Autodesk Fusion 360 part; units mm, degrees
note: some values were not read from the file. Chosen so that the rebuilt part matches the saved one: which bodies a step acts on; which face or edge a step refers to. Set by a fixed rule: which sketch regions a step uses.
(part 2 of 2)
sketch "Sketch5" plane through (0, 0, 0) normal (0, 0, 1) x (-1, 0, 0)
  line L0 (-11.6608, -63.9455) -> (-11.5909, -63.4815)
  line L1 (-11.5909, -63.4815) -> (-7.6356, -64.0777)
  line L2 (-7.6356, -64.0777) -> (-7.7055, -64.5417)
  arc A0 (-7.7055, -64.5417) -> (-2, -64.9692) centre (0, 0) ccw
  line L3 (-2, -64.9692) -> (-2, -64.5)
  line L4 (-2, -64.5) -> (2, -64.5)
  line L5 (2, -64.5) -> (2, -64.9692)
  arc A1 (2, -64.9692) -> (7.7055, -64.5417) centre (0, 0) ccw
  line L6 (7.7055, -64.5417) -> (7.6356, -64.0777)
  line L7 (7.6356, -64.0777) -> (11.5909, -63.4815)
  line L8 (11.5909, -63.4815) -> (11.6608, -63.9455)
  arc A2 (11.6608, -63.9455) -> (17.2389, -62.6723) centre (0, 0) ccw
  line L9 (17.2389, -62.6723) -> (17.1006, -62.224)
  line L10 (17.1006, -62.224) -> (20.9229, -61.0449)
  line L11 (20.9229, -61.0449) -> (21.0612, -61.4933)
  arc A3 (21.0612, -61.4933) -> (26.3872, -59.403) centre (0, 0) ccw
  line L12 (26.3872, -59.403) -> (26.1836, -58.9803)
  line L13 (26.1836, -58.9803) -> (29.7874, -57.2447)
  line L14 (29.7874, -57.2447) -> (29.991, -57.6675)
  arc A4 (29.991, -57.6675) -> (34.946, -54.8067) centre (0, 0) ccw
  line L15 (34.946, -54.8067) -> (34.6817, -54.419)
  line L16 (34.6817, -54.419) -> (37.9866, -52.1658)
  line L17 (37.9866, -52.1658) -> (38.2509, -52.5535)
  arc A5 (38.2509, -52.5535) -> (42.7242, -48.9862) centre (0, 0) ccw
  line L18 (42.7242, -48.9862) -> (42.405, -48.6422)
  line L19 (42.405, -48.6422) -> (45.3372, -45.9215)
  line L20 (45.3372, -45.9215) -> (45.6564, -46.2655)
  arc A6 (45.6564, -46.2655) -> (49.548, -42.0713) centre (0, 0) ccw
  line L21 (49.548, -42.0713) -> (49.1812, -41.7788)
  line L22 (49.1812, -41.7788) -> (51.6751, -38.6514)
  line L23 (51.6751, -38.6514) -> (52.042, -38.944)
  arc A7 (52.042, -38.944) -> (55.265, -34.2167) centre (0, 0) ccw
  line L24 (55.265, -34.2167) -> (54.8586, -33.9821)
  line L25 (54.8586, -33.9821) -> (56.8586, -30.5179)
  line L26 (56.8586, -30.5179) -> (57.265, -30.7526)
  arc A8 (57.265, -30.7526) -> (59.7475, -25.5977) centre (0, 0) ccw
  line L27 (59.7475, -25.5977) -> (59.3107, -25.4262)
  line L28 (59.3107, -25.4262) -> (60.772, -21.7027)
  line L29 (60.772, -21.7027) -> (61.2088, -21.8742)
  arc A9 (61.2088, -21.8742) -> (62.8953, -16.4069) centre (0, 0) ccw
  line L30 (62.8953, -16.4069) -> (62.4378, -16.3025)
  line L31 (62.4378, -16.3025) -> (63.3279, -12.4027)
  line L32 (63.3279, -12.4027) -> (63.7854, -12.5072)
  arc A10 (63.7854, -12.5072) -> (64.6381, -6.8496) centre (0, 0) ccw
  line L33 (64.6381, -6.8496) -> (64.1702, -6.8145)
  line L34 (64.1702, -6.8145) -> (64.4691, -2.8257)
  line L35 (64.4691, -2.8257) -> (64.937, -2.8607)
  arc A11 (64.937, -2.8607) -> (64.937, 2.8607) centre (0, 0) ccw
  line L36 (64.937, 2.8607) -> (64.4691, 2.8257)
  line L37 (64.4691, 2.8257) -> (64.1702, 6.8145)
  line L38 (64.1702, 6.8145) -> (64.6381, 6.8496)
  arc A12 (64.6381, 6.8496) -> (63.7854, 12.5072) centre (0, 0) ccw
  line L39 (63.7854, 12.5072) -> (63.3279, 12.4027)
  line L40 (63.3279, 12.4027) -> (62.4378, 16.3025)
  line L41 (62.4378, 16.3025) -> (62.8953, 16.4069)
  arc A13 (62.8953, 16.4069) -> (61.2088, 21.8742) centre (0, 0) ccw
  line L42 (61.2088, 21.8742) -> (60.772, 21.7027)
  line L43 (60.772, 21.7027) -> (59.3107, 25.4262)
  line L44 (59.3107, 25.4262) -> (59.7475, 25.5977)
  arc A14 (59.7475, 25.5977) -> (57.265, 30.7526) centre (0, 0) ccw
  line L45 (57.265, 30.7526) -> (56.8586, 30.5179)
  line L46 (56.8586, 30.5179) -> (54.8586, 33.9821)
  line L47 (54.8586, 33.9821) -> (55.265, 34.2167)
  arc A15 (55.265, 34.2167) -> (52.042, 38.944) centre (0, 0) ccw
  line L48 (52.042, 38.944) -> (51.6751, 38.6514)
  line L49 (51.6751, 38.6514) -> (49.1812, 41.7788)
  line L50 (49.1812, 41.7788) -> (49.548, 42.0713)
  arc A16 (49.548, 42.0713) -> (45.6564, 46.2655) centre (0, 0) ccw
  line L51 (45.6564, 46.2655) -> (45.3372, 45.9215)
  line L52 (45.3372, 45.9215) -> (42.405, 48.6422)
  line L53 (42.405, 48.6422) -> (42.7242, 48.9862)
  arc A17 (42.7242, 48.9862) -> (38.2509, 52.5535) centre (0, 0) ccw
  line L54 (38.2509, 52.5535) -> (37.9866, 52.1658)
  line L55 (37.9866, 52.1658) -> (34.6817, 54.419)
  line L56 (34.6817, 54.419) -> (34.946, 54.8067)
  arc A18 (34.946, 54.8067) -> (29.991, 57.6675) centre (0, 0) ccw
  line L57 (29.991, 57.6675) -> (29.7874, 57.2447)
  line L58 (29.7874, 57.2447) -> (26.1836, 58.9803)
  line L59 (26.1836, 58.9803) -> (26.3872, 59.403)
  arc A19 (26.3872, 59.403) -> (21.0612, 61.4933) centre (0, 0) ccw
  line L60 (21.0612, 61.4933) -> (20.9229, 61.0449)
  line L61 (20.9229, 61.0449) -> (17.1006, 62.224)
  line L62 (17.1006, 62.224) -> (17.2389, 62.6723)
  arc A20 (17.2389, 62.6723) -> (11.6608, 63.9455) centre (0, 0) ccw
  line L63 (11.6608, 63.9455) -> (11.5909, 63.4815)
  line L64 (11.5909, 63.4815) -> (7.6356, 64.0777)
  line L65 (7.6356, 64.0777) -> (7.7055, 64.5417)
  arc A21 (7.7055, 64.5417) -> (2, 64.9692) centre (0, 0) ccw
  line L66 (2, 64.9692) -> (2, 64.5)
  line L67 (2, 64.5) -> (-2, 64.5)
  line L68 (-2, 64.5) -> (-2, 64.9692)
  arc A22 (-2, 64.9692) -> (-7.7055, 64.5417) centre (0, 0) ccw
  line L69 (-7.7055, 64.5417) -> (-7.6356, 64.0777)
  line L70 (-7.6356, 64.0777) -> (-11.5909, 63.4815)
  line L71 (-11.5909, 63.4815) -> (-11.6608, 63.9455)
  arc A23 (-11.6608, 63.9455) -> (-17.2389, 62.6723) centre (0, 0) ccw
  line L72 (-17.2389, 62.6723) -> (-17.1006, 62.224)
  line L73 (-17.1006, 62.224) -> (-20.9229, 61.0449)
  line L74 (-20.9229, 61.0449) -> (-21.0612, 61.4933)
  arc A24 (-21.0612, 61.4933) -> (-26.3872, 59.403) centre (0, 0) ccw
  line L75 (-26.3872, 59.403) -> (-26.1836, 58.9803)
  line L76 (-26.1836, 58.9803) -> (-29.7874, 57.2447)
  line L77 (-29.7874, 57.2447) -> (-29.991, 57.6675)
  arc A25 (-29.991, 57.6675) -> (-34.946, 54.8067) centre (0, 0) ccw
  line L78 (-34.946, 54.8067) -> (-34.6817, 54.419)
  line L79 (-34.6817, 54.419) -> (-37.9866, 52.1658)
  line L80 (-37.9866, 52.1658) -> (-38.2509, 52.5535)
  arc A26 (-38.2509, 52.5535) -> (-42.7242, 48.9862) centre (0, 0) ccw
  line L81 (-42.7242, 48.9862) -> (-42.405, 48.6422)
  line L82 (-42.405, 48.6422) -> (-45.3372, 45.9215)
  line L83 (-45.3372, 45.9215) -> (-45.6564, 46.2655)
  arc A27 (-45.6564, 46.2655) -> (-49.548, 42.0713) centre (0, 0) ccw
  line L84 (-49.548, 42.0713) -> (-49.1812, 41.7788)
  line L85 (-49.1812, 41.7788) -> (-51.6751, 38.6514)
  line L86 (-51.6751, 38.6514) -> (-52.042, 38.944)
  arc A28 (-52.042, 38.944) -> (-55.265, 34.2167) centre (0, 0) ccw
  line L87 (-55.265, 34.2167) -> (-54.8586, 33.9821)
  line L88 (-54.8586, 33.9821) -> (-56.8586, 30.5179)
  line L89 (-56.8586, 30.5179) -> (-57.265, 30.7526)
  arc A29 (-57.265, 30.7526) -> (-59.7475, 25.5977) centre (0, 0) ccw
  line L90 (-59.7475, 25.5977) -> (-59.3107, 25.4262)
  line L91 (-59.3107, 25.4262) -> (-60.772, 21.7027)
  line L92 (-60.772, 21.7027) -> (-61.2088, 21.8742)
  arc A30 (-61.2088, 21.8742) -> (-62.8953, 16.4069) centre (0, 0) ccw
  line L93 (-62.8953, 16.4069) -> (-62.4378, 16.3025)
  line L94 (-62.4378, 16.3025) -> (-63.3279, 12.4027)
  line L95 (-63.3279, 12.4027) -> (-63.7854, 12.5072)
  arc A31 (-63.7854, 12.5072) -> (-64.6381, 6.8496) centre (0, 0) ccw
  line L96 (-64.6381, 6.8496) -> (-64.1702, 6.8145)
  line L97 (-64.1702, 6.8145) -> (-64.4691, 2.8257)
  line L98 (-64.4691, 2.8257) -> (-64.937, 2.8607)
  arc A32 (-64.937, 2.8607) -> (-64.937, -2.8607) centre (0, 0) ccw
  line L99 (-64.937, -2.8607) -> (-64.4691, -2.8257)
  line L100 (-64.4691, -2.8257) -> (-64.1702, -6.8145)
  line L101 (-64.1702, -6.8145) -> (-64.6381, -6.8496)
  arc A33 (-64.6381, -6.8496) -> (-63.7854, -12.5072) centre (0, 0) ccw
  line L102 (-63.7854, -12.5072) -> (-63.3279, -12.4027)
  line L103 (-63.3279, -12.4027) -> (-62.4378, -16.3025)
  line L104 (-62.4378, -16.3025) -> (-62.8953, -16.4069)
  arc A34 (-62.8953, -16.4069) -> (-61.2088, -21.8742) centre (0, 0) ccw
  line L105 (-61.2088, -21.8742) -> (-60.772, -21.7027)
  line L106 (-60.772, -21.7027) -> (-59.3107, -25.4262)
  line L107 (-59.3107, -25.4262) -> (-59.7475, -25.5977)
  arc A35 (-59.7475, -25.5977) -> (-57.265, -30.7526) centre (0, 0) ccw
  line L108 (-57.265, -30.7526) -> (-56.8586, -30.5179)
  line L109 (-56.8586, -30.5179) -> (-54.8586, -33.9821)
  line L110 (-54.8586, -33.9821) -> (-55.265, -34.2167)
  arc A36 (-55.265, -34.2167) -> (-52.042, -38.944) centre (0, 0) ccw
  line L111 (-52.042, -38.944) -> (-51.6751, -38.6514)
  line L112 (-51.6751, -38.6514) -> (-49.1812, -41.7788)
  line L113 (-49.1812, -41.7788) -> (-49.548, -42.0713)
  arc A37 (-49.548, -42.0713) -> (-45.6564, -46.2655) centre (0, 0) ccw
  line L114 (-45.6564, -46.2655) -> (-45.3372, -45.9215)
  line L115 (-45.3372, -45.9215) -> (-42.405, -48.6422)
  line L116 (-42.405, -48.6422) -> (-42.7242, -48.9862)
  arc A38 (-42.7242, -48.9862) -> (-38.2509, -52.5535) centre (0, 0) ccw
  line L117 (-38.2509, -52.5535) -> (-37.9866, -52.1658)
  line L118 (-37.9866, -52.1658) -> (-34.6817, -54.419)
  line L119 (-34.6817, -54.419) -> (-34.946, -54.8067)
  arc A39 (-34.946, -54.8067) -> (-29.991, -57.6675) centre (0, 0) ccw
  line L120 (-29.991, -57.6675) -> (-29.7874, -57.2447)
  line L121 (-29.7874, -57.2447) -> (-26.1836, -58.9803)
  line L122 (-26.1836, -58.9803) -> (-26.3872, -59.403)
  arc A40 (-26.3872, -59.403) -> (-21.0612, -61.4933) centre (0, 0) ccw
  line L123 (-21.0612, -61.4933) -> (-20.9229, -61.0449)
  line L124 (-20.9229, -61.0449) -> (-17.1006, -62.224)
  line L125 (-17.1006, -62.224) -> (-17.2389, -62.6723)
  arc A41 (-17.2389, -62.6723) -> (-11.6608, -63.9455) centre (0, 0) ccw
  arc A42 (44.2503, 36.7173) -> (-44.2503, 36.7173) centre (0, 0) ccw
  arc A43 (43.1721, 30.6989) -> (44.2503, 36.7173) centre (41.1721, 34.163) ccw
  line L126 (43.1721, 30.6989) -> (23.6426, 19.4236)
  arc A44 (18.8944, 19.9813) -> (23.6426, 19.4236) centre (21.6426, 22.8877) ccw
  arc A45 (18.8944, 19.9813) -> (-18.8944, 19.9813) centre (0, 0) ccw
  arc A46 (-23.6426, 19.4236) -> (-18.8944, 19.9813) centre (-21.6426, 22.8877) ccw
  line L127 (-23.6426, 19.4236) -> (-43.1721, 30.6989)
  arc A47 (-44.2503, 36.7173) -> (-43.1721, 30.6989) centre (-41.1721, 34.163) ccw
  arc A48 (-26.7515, 6.3723) -> (-7.8571, -26.3537) centre (0, 0) ccw
  arc A49 (-5, -30.1869) -> (-7.8571, -26.3537) centre (-9, -30.1869) ccw
  line L128 (-5, -30.1869) -> (-5, -52.7376)
  arc A50 (-9.6729, -56.6806) -> (-5, -52.7376) centre (-9, -52.7376) ccw
  arc A51 (-53.9232, 19.9633) -> (-9.6729, -56.6806) centre (0, 0) ccw
  arc A52 (-48.1721, 22.0387) -> (-53.9232, 19.9633) centre (-50.1721, 18.5746) ccw
  line L129 (-48.1721, 22.0387) -> (-28.6426, 10.7633)
  arc A53 (-26.7515, 6.3723) -> (-28.6426, 10.7633) centre (-30.6426, 7.2992) ccw
  line L130 (-2.3412, -7.1252) -> (-9.1913, -11.0801)
  arc A54 (-14.6554, -9.616) -> (-9.1913, -11.0801) centre (-11.1913, -7.616) ccw
  line L131 (-14.6554, -9.616) -> (-15.6554, -7.884)
  arc A55 (-14.1913, -2.4199) -> (-15.6554, -7.884) centre (-12.1913, -5.884) ccw
  line L132 (-14.1913, -2.4199) -> (-7.3412, 1.535)
  arc A56 (-5, 5.5902) -> (-7.3412, 1.535) centre (0, 0) ccw
  line L133 (-5, 5.5902) -> (-5, 13.5)
  arc A57 (-1, 17.5) -> (-5, 13.5) centre (-1, 13.5) ccw
  line L134 (-1, 17.5) -> (1, 17.5)
  arc A58 (5, 13.5) -> (1, 17.5) centre (1, 13.5) ccw
  line L135 (5, 13.5) -> (5, 5.5902)
  arc A59 (7.3412, 1.535) -> (5, 5.5902) centre (0, 0) ccw
  line L136 (7.3412, 1.535) -> (14.1913, -2.4199)
  arc A60 (15.6554, -7.884) -> (14.1913, -2.4199) centre (12.1913, -5.884) ccw
  line L137 (15.6554, -7.884) -> (14.6554, -9.616)
  arc A61 (9.1913, -11.0801) -> (14.6554, -9.616) centre (11.1913, -7.616) ccw
  line L138 (9.1913, -11.0801) -> (2.3412, -7.1252)
  arc A62 (-2.3412, -7.1252) -> (2.3412, -7.1252) centre (0, 0) ccw
  arc A63 (7.8571, -26.3537) -> (26.7515, 6.3723) centre (0, 0) ccw
  arc A64 (28.6426, 10.7633) -> (26.7515, 6.3723) centre (30.6426, 7.2992) ccw
  line L139 (28.6426, 10.7633) -> (48.1721, 22.0387)
  arc A65 (53.9232, 19.9633) -> (48.1721, 22.0387) centre (50.1721, 18.5746) ccw
  arc A66 (9.6729, -56.6806) -> (53.9232, 19.9633) centre (0, 0) ccw
  arc A67 (5, -52.7376) -> (9.6729, -56.6806) centre (9, -52.7376) ccw
  line L140 (5, -52.7376) -> (5, -30.1869)
  arc A68 (7.8571, -26.3537) -> (5, -30.1869) centre (9, -30.1869) ccw

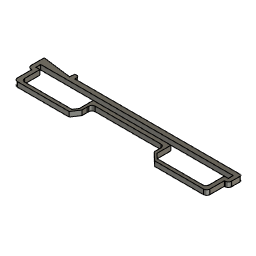
design "Dual Dc and gear"
Autodesk Fusion 360 part; units mm, degrees
sketch "Sketch1" plane through (0, 0, 0) normal (0, 0, 1) x (1, 0, 0)
  line L0 (-83.1348, 11.7496) -> (-83.1348, 16.7496)
  line L1 (-48.4171, -17.3931) -> (-51.4981, -22.0146)
  line L2 (45, -5) -> (45, -17.3931)
  line L3 (-51.4981, -22.0146) -> (-115, -22.0146)
  line L4 (48.3777, -17.3931) -> (48.3777, 0)
  line L5 (55, -27) -> (120, -27)
  line L6 (-115, 0) -> (-120, 0)
  line L7 (-120, 0) -> (-120, 6)
  line L8 (-120, 6) -> (120, 6)
  line L9 (48.3777, 0) -> (-48.4171, 0)
  line L10 (115, -22.0146) -> (53.2559, -22.0146)
  line L11 (53.2559, -22.0146) -> (48.3777, -17.3931)
  line L12 (-88.9, 10.8) -> (-120, 14.8)
  line L13 (125, 11.7496) -> (-83.1348, 11.7496)
  line L14 (-45, -5) -> (45, -5)
  line L15 (-115, -22.0146) -> (-115, 0)
  line L16 (-120, -5) -> (-120, -27.0146)
  line L17 (-48.4171, 0) -> (-48.4171, -17.3931)
  line L18 (-88.1348, 16.7496) -> (-88.9, 10.8)
  line L19 (-45.0838, -17.3931) -> (-45.0838, -11)
  line L20 (-125.0002, -5) -> (-120, -5)
  line L21 (120, -5) -> (125, -5)
  line L22 (120, -27) -> (120, -5)
  line L23 (53.2559, -25.2145) -> (55, -27)
  line L24 (125, -5) -> (125, 11.7496)
  line L25 (-51.4981, -27.0146) -> (-45.0838, -17.3931)
  line L26 (-45.0838, -11) -> (-45, -5)
  line L27 (-120, -27.0146) -> (-51.4981, -27.0146)
  line L28 (-125.0002, 15.4377) -> (-125.0002, -5)
  line L29 (115, 0) -> (115, -22.0146)
  line L30 (-83.1348, 16.7496) -> (-88.1348, 16.7496)
  line L31 (120, 6) -> (120, 0)
  line L32 (-120, 14.8) -> (-125.0002, 15.4377)
  line L33 (45, -17.3931) -> (53.2559, -25.2145)
  line L34 (120, 0) -> (115, 0)
extrude "Extrude1" add sketch "Sketch1" along normal blind 6
fillet "Fillet1" radius 4 6 edges at (120, -27, 3) (125, -5, 3) (45, -5, 3) (-45, -5, 3) (-120, -27.0146, 3) (-125.0002, -5, 3)
sketch "Sketch2" plane through (0, 0, 6) normal (0, 0, 1) x (-1, 0, 0)
  arc A0 (125.0002, 1) -> (121.0002, 5) centre (121.0002, 1) ccw
  line L0 (121.0002, 5) -> (120, 5)
  line L1 (120, 5) -> (120, 23.0146)
  arc A1 (120, 23.0146) -> (116, 27.0146) centre (116, 23.0146) ccw
  line L2 (116, 27.0146) -> (51.4981, 27.0146)
  line L3 (51.4981, 27.0146) -> (45.0838, 17.3931)
  line L4 (45.0838, 17.3931) -> (45.0838, 11)
  line L5 (45.0838, 11) -> (45.0551, 8.9442)
  arc A2 (41.0555, 5) -> (45.0551, 8.9442) centre (41.0555, 9) ccw
  line L6 (41.0555, 5) -> (-41, 5)
  arc A3 (-45, 9) -> (-41, 5) centre (-41, 9) ccw
  line L7 (-45, 9) -> (-45, 17.3931)
  line L8 (-45, 17.3931) -> (-53.2559, 25.2145)
  line L9 (-53.2559, 25.2145) -> (-55, 27)
  line L10 (-55, 27) -> (-116, 27)
  arc A4 (-116, 27) -> (-120, 23) centre (-116, 23) ccw
  line L11 (-120, 23) -> (-120, 5)
  line L12 (-120, 5) -> (-121, 5)
  arc A5 (-121, 5) -> (-125, 1) centre (-121, 1) ccw
  line L13 (-125, 1) -> (-125, -11.7496)
  line L14 (-125, -11.7496) -> (83.1348, -11.7496)
  line L15 (83.1348, -11.7496) -> (83.1348, -16.7496)
  line L16 (83.1348, -16.7496) -> (88.1348, -16.7496)
  line L17 (88.1348, -16.7496) -> (88.9, -10.8)
  line L18 (88.9, -10.8) -> (120, -14.8)
  line L19 (120, -14.8) -> (125.0002, -15.4377)
  line L20 (125.0002, -15.4377) -> (125.0002, 1)
  line L21 (-120, -6) -> (-120, 0)
  line L22 (-120, 0) -> (-115, 0)
  line L23 (-115, 0) -> (-115, 22.0146)
  line L24 (-115, 22.0146) -> (-53.2559, 22.0146)
  line L25 (-53.2559, 22.0146) -> (-48.3777, 17.3931)
  line L26 (-48.3777, 17.3931) -> (-48.3777, 0)
  line L27 (-48.3777, 0) -> (48.4171, 0)
  line L28 (48.4171, 0) -> (48.4171, 17.3931)
  line L29 (48.4171, 17.3931) -> (51.4981, 22.0146)
  line L30 (51.4981, 22.0146) -> (115, 22.0146)
  line L31 (115, 22.0146) -> (115, 0)
  line L32 (115, 0) -> (120, 0)
  line L33 (120, 0) -> (120, -6)
  line L34 (120, -6) -> (-120, -6)
  line L35 (-115, 22.0146) -> (-115, 23.0146)
  line L36 (-115, 23.0146) -> (-54.3115, 23.0146)
  line L37 (-54.3115, 23.0146) -> (-53.2559, 22.0146)
  dimension "d7" = 1
  constraint coincident L23.end L24.start
  constraint perpendicular L24 L35
  constraint perpendicular L35 L36
  constraint coincident L24.end L25.start
  constraint parallel L25 L37
  measures "d7" distance of L23.end L35.end
extrude "Extrude2" cut sketch "Sketch2" against normal blind 14 contours L24 L35 L36 L37
fillet "Fillet3" radius 4 1 edges at (115, -23.0146, 3)
sketch "Sketch3" plane through (0, 0, 6) normal (0, 0, 1) x (-1, 0, 0)
  line L0 (-115, 0) -> (-115, 19.0146)
  arc A0 (-111, 23.0146) -> (-115, 19.0146) centre (-111, 19.0146) ccw
  line L1 (-111, 23.0146) -> (-54.3115, 23.0146)
  line L2 (-54.3115, 23.0146) -> (-48.3777, 17.3931)
  line L3 (-48.3777, 17.3931) -> (-48.3777, 0)
  line L4 (-48.3777, 0) -> (48.4171, 0)
  line L5 (48.4171, 0) -> (48.4171, 17.3931)
  line L6 (48.4171, 17.3931) -> (51.4981, 22.0146)
  line L7 (51.4981, 22.0146) -> (115, 22.0146)
  line L8 (115, 22.0146) -> (115, 0)
  line L9 (115, 0) -> (120, 0)
  line L10 (120, 0) -> (120, -6)
  line L11 (120, -6) -> (-120, -6)
  line L12 (-120, -6) -> (-120, 0)
  line L13 (-120, 0) -> (-115, 0)
  arc A1 (125.0002, 1) -> (121.0002, 5) centre (121.0002, 1) ccw
  line L14 (121.0002, 5) -> (120, 5)
  line L15 (120, 5) -> (120, 23.0146)
  arc A2 (120, 23.0146) -> (116, 27.0146) centre (116, 23.0146) ccw
  line L16 (116, 27.0146) -> (51.4981, 27.0146)
  line L17 (51.4981, 27.0146) -> (45.0838, 17.3931)
  line L18 (45.0838, 17.3931) -> (45.0838, 11)
  line L19 (45.0838, 11) -> (45.0551, 8.9442)
  arc A3 (41.0555, 5) -> (45.0551, 8.9442) centre (41.0555, 9) ccw
  line L20 (41.0555, 5) -> (-41, 5)
  arc A4 (-45, 9) -> (-41, 5) centre (-41, 9) ccw
  line L21 (-45, 9) -> (-45, 17.3931)
  line L22 (-45, 17.3931) -> (-53.2559, 25.2145)
  line L23 (-53.2559, 25.2145) -> (-55, 27)
  line L24 (-55, 27) -> (-116, 27)
  arc A5 (-116, 27) -> (-120, 23) centre (-116, 23) ccw
  line L25 (-120, 23) -> (-120, 5)
  line L26 (-120, 5) -> (-121, 5)
  arc A6 (-121, 5) -> (-125, 1) centre (-121, 1) ccw
  line L27 (-125, 1) -> (-125, -11.7496)
  line L28 (-125, -11.7496) -> (83.1348, -11.7496)
  line L29 (83.1348, -11.7496) -> (83.1348, -16.7496)
  line L30 (83.1348, -16.7496) -> (88.1348, -16.7496)
  line L31 (88.1348, -16.7496) -> (88.9, -10.8)
  line L32 (88.9, -10.8) -> (120, -14.8)
  line L33 (120, -14.8) -> (125.0002, -15.4377)
  line L34 (125.0002, -15.4377) -> (125.0002, 1)
  line L35 (115, 22.0146) -> (115, 23.0146)
  line L36 (115, 23.0146) -> (52.1648, 23.0146)
  line L37 (52.1648, 23.0146) -> (51.4981, 22.0146)
  dimension "d12" = 1
  constraint coincident L7.end L8.start
  constraint perpendicular L7 L35
  constraint perpendicular L8 L36
  constraint coincident L6.end L7.start
  constraint parallel L6 L37
  measures "d12" distance of L7.end L35.end
extrude "Extrude3" cut sketch "Sketch3" against normal blind 12 contours L7 L35 L36 L37
fillet "Fillet4" radius 4 1 edges at (-115, -23.0146, 3)
fillet "Fillet5" radius 2 1 edges at (125, 11.7496, 3)
fillet "Fillet6" radius 2 1 edges at (-83.1348, 16.7496, 3)
fillet "Fillet7" radius 1 1 edges at (115, 0, 3)
sketch "Sketch4" plane through (0, 0, 6) normal (0, 0, 1) x (-1, 0, 0)
  arc A0 (-116, 0) -> (-115, 1) centre (-116, 1) ccw
  line L0 (-115, 1) -> (-115, 19.0146)
  arc A1 (-111, 23.0146) -> (-115, 19.0146) centre (-111, 19.0146) ccw
  line L1 (-111, 23.0146) -> (-54.3115, 23.0146)
  line L2 (-54.3115, 23.0146) -> (-48.3777, 17.3931)
  line L3 (-48.3777, 17.3931) -> (-48.3777, 0)
  line L4 (-48.3777, 0) -> (48.4171, 0)
  line L5 (48.4171, 0) -> (48.4171, 17.3931)
  line L6 (48.4171, 17.3931) -> (52.1648, 23.0146)
  line L7 (52.1648, 23.0146) -> (111, 23.0146)
  arc A2 (115, 19.0146) -> (111, 23.0146) centre (111, 19.0146) ccw
  line L8 (115, 19.0146) -> (115, 0)
  line L9 (115, 0) -> (120, 0)
  line L10 (120, 0) -> (120, -6)
  line L11 (120, -6) -> (-120, -6)
  line L12 (-120, -6) -> (-120, 0)
  line L13 (-120, 0) -> (-116, 0)
  arc A3 (83.1348, -14.7496) -> (85.1348, -16.7496) centre (85.1348, -14.7496) ccw
  line L14 (85.1348, -16.7496) -> (88.1348, -16.7496)
  line L15 (88.1348, -16.7496) -> (88.9, -10.8)
  line L16 (88.9, -10.8) -> (120, -14.8)
  line L17 (120, -14.8) -> (125.0002, -15.4377)
  line L18 (125.0002, -15.4377) -> (125.0002, 1)
  arc A4 (125.0002, 1) -> (121.0002, 5) centre (121.0002, 1) ccw
  line L19 (121.0002, 5) -> (120, 5)
  line L20 (120, 5) -> (120, 23.0146)
  arc A5 (120, 23.0146) -> (116, 27.0146) centre (116, 23.0146) ccw
  line L21 (116, 27.0146) -> (51.4981, 27.0146)
  line L22 (51.4981, 27.0146) -> (45.0838, 17.3931)
  line L23 (45.0838, 17.3931) -> (45.0838, 11)
  line L24 (45.0838, 11) -> (45.0551, 8.9442)
  arc A6 (41.0555, 5) -> (45.0551, 8.9442) centre (41.0555, 9) ccw
  line L25 (41.0555, 5) -> (-41, 5)
  arc A7 (-45, 9) -> (-41, 5) centre (-41, 9) ccw
  line L26 (-45, 9) -> (-45, 17.3931)
  line L27 (-45, 17.3931) -> (-53.2559, 25.2145)
  line L28 (-53.2559, 25.2145) -> (-55, 27)
  line L29 (-55, 27) -> (-116, 27)
  arc A8 (-116, 27) -> (-120, 23) centre (-116, 23) ccw
  line L30 (-120, 23) -> (-120, 5)
  line L31 (-120, 5) -> (-121, 5)
  arc A9 (-121, 5) -> (-125, 1) centre (-121, 1) ccw
  line L32 (-125, 1) -> (-125, -9.7496)
  arc A10 (-125, -9.7496) -> (-123, -11.7496) centre (-123, -9.7496) ccw
  line L33 (-123, -11.7496) -> (83.1348, -11.7496)
  line L34 (83.1348, -11.7496) -> (83.1348, -14.7496)

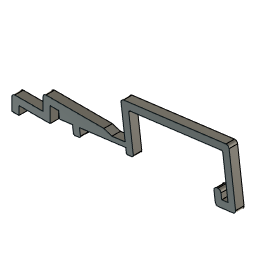
design "HOOK ARM"
Autodesk Fusion 360 part; units mm, degrees
ref_plane "WorkPlane1" through (112.1576, 66, 17) normal (0, 1, 0) x (-1, 0, 0)
sketch "Sketch2" plane through (0, 66, 0) normal (0, 1, 0) x (1, 0, 0)
  line L0 (87, -6) -> (87, -28)
  line L1 (87, -28) -> (130, -28)
  line L2 (130, -28) -> (136, -26)
  line L3 (136, -26) -> (137, -23)
  line L4 (137, -23) -> (98, -18)
  line L5 (98, -18) -> (98, -23)
  line L6 (98, -23) -> (92, -23)
  line L7 (92, -23) -> (92, -6)
  line L8 (92, -6) -> (87, -6)
  constraint vertical L0
  constraint perpendicular L0 L1
  constraint perpendicular L1 L5
  constraint perpendicular L5 L6
  constraint perpendicular L6 L7
  constraint perpendicular L7 L8
extrude "Extrude1" add sketch "Sketch2" along normal blind 6 makes body 1
sketch "Sketch3" plane through (-0.6856, 0, 5.348) normal (0.127164, 0, -0.991882) x (0, 1, 0)
  line L0 (66, 138.8126) -> (66, 99.4934)
  line L1 (66, 99.4934) -> (72, 99.4934)
  line L2 (72, 99.4934) -> (72, 138.8126)
  line L3 (72, 138.8126) -> (66, 138.8126)
  line L4 (69.556, 99.4934) -> (69.556, 104.3824) construction
  line L5 (72, 104.3824) -> (66, 104.3824)
  line L6 (66, 104.3824) -> (66, 109.3824)
  line L7 (66, 109.3824) -> (72, 109.3824)
  line L8 (72, 109.3824) -> (72, 104.3824)
  line L9 (72, 109.3824) -> (66, 109.3824)
  line L10 (66, 109.3824) -> (66, 114.3824)
  line L11 (66, 114.3824) -> (72, 114.3824)
  line L12 (72, 114.3824) -> (72, 109.3824)
  dimension "d4" = 4.889
  dimension "d5" = 5
  dimension "d46" = 5
  constraint coincident L1 L4.start
  constraint perpendicular L1 L4
  constraint horizontal L5
  constraint vertical L6
  constraint horizontal L7
  constraint vertical L8
  constraint coincident L2 L5.start
  constraint horizontal L9
  constraint vertical L10
  constraint horizontal L11
  constraint vertical L12
  constraint coincident L0 L10.end
  measures "d4" distance of L4.start L4.end
  measures "d5" distance of L5.start L7.end
  measures "d46" distance of L7.end L11.end
sketch "Sketch4" plane through (0, 72, 0) normal (0, 1, 0) x (-1, 0, 0)
  line L0 (-137, 23) -> (-98, 18)
  line L1 (-98, 18) -> (-98, 23)
  line L2 (-98, 23) -> (-92, 23)
  line L3 (-92, 23) -> (-92, 6)
  line L4 (-92, 6) -> (-87, 6)
  line L5 (-87, 6) -> (-87, 28)
  line L6 (-87, 28) -> (-130, 28)
  line L7 (-130, 28) -> (-136, 26)
  line L8 (-136, 26) -> (-137, 23)
  line L9 (-87, 6) -> (-92, 6)
  line L10 (-92, 6) -> (-92, 12)
  line L11 (-92, 12) -> (-87, 12)
  line L12 (-87, 12) -> (-87, 6)
  line L13 (-87, 12) -> (-65, 12)
  line L14 (-65, 6) -> (-65, 12)
  line L15 (-65, 17) -> (-87, 17)
  line L16 (-65, 6) -> (-70, 6)
  line L17 (-70, 6) -> (-70, 12)
  line L18 (-70, 12) -> (-65, 12)
  line L19 (-65, 12) -> (-65, 6)
  line L20 (-65, 12) -> (-65, 17)
  constraint horizontal L9
  constraint vertical L10
  constraint horizontal L11
  constraint vertical L12
  constraint coincident L3 L10.end
  constraint coincident L4.end L5.start
  constraint perpendicular L5 L13
  constraint perpendicular L13 L14
  constraint midpoint L5 L15.end
  constraint perpendicular L5 L15
  constraint horizontal L16
  constraint vertical L17
  constraint horizontal L18
  constraint vertical L19
  constraint coincident L13 L17.end
  constraint perpendicular L18 L20
extrude "Extrude3" cut sketch "Sketch4" against normal blind 6.5 contours L3 L4 L5 L9 L10 L11 L12 bodies 1
extrude "Extrude4" add sketch "Sketch4" against normal blind 6 contours L5 L13 L15 L18 L20 | L13 L14 L16 L17 L18 L19 bodies 1
sketch "Sketch5" plane through (-0.6856, 0, 5.348) normal (0.127164, 0, -0.991882) x (0, 1, 0)
  line L0 (72, 99.4934) -> (72, 138.8126)
  line L1 (72, 138.8126) -> (66, 138.8126)
  line L2 (66, 138.8126) -> (66, 99.4934)
  line L3 (69, 109.3824) -> (69, 147.2714) construction
  line L4 (69, 147.2714) -> (66, 147.2714) construction
  line L5 (66, 147.2714) -> (66, 144.7714) construction
  line L6 (66, 144.7714) -> (69, 144.7714) construction
  line L7 (69, 144.7714) -> (69, 147.2714) construction
  line L8 (66, 144.7714) -> (72, 144.7714)
  line L9 (72, 144.7714) -> (72, 149.7714)
  line L10 (72, 149.7714) -> (66, 149.7714)
  line L11 (66, 149.7714) -> (66, 144.7714)
  line L12 (66, 99.4934) -> (72, 99.4934)
  dimension "d21" = 37.889
  dimension "d22" = 2.5
  dimension "d23" = 5
  constraint perpendicular L1 L3
  constraint horizontal L4
  constraint vertical L5
  constraint horizontal L6
  constraint vertical L7
  constraint horizontal L8
  constraint vertical L9
  constraint horizontal L10
  constraint vertical L11
  measures "d21" distance of L3.start L3.end
  measures "d22" distance of L3.end L6.end
  measures "d23" distance of L5.end L10.end
sketch "Sketch6" plane through (0, 66, 0) normal (0, -1, 0) x (1, 0, 0)
  line L0 (65, 17) -> (65, 6)
  line L1 (70, 12) -> (92, 12)
  line L2 (92, 12) -> (92, 23)
  line L3 (92, 23) -> (98, 23)
  line L4 (98, 23) -> (98, 18)
  line L5 (98, 18) -> (137, 23)
  line L6 (137, 23) -> (136, 26)
  line L7 (136, 26) -> (130, 28)
  line L8 (130, 28) -> (87, 28)
  line L9 (87, 28) -> (87, 17)
  line L10 (87, 17) -> (65, 17)
  line L11 (136.0676, 22.8805) -> (135.6529, 26.1157)
  line L12 (65, 6) -> (70, 6)
  line L13 (70, 6) -> (70, 12)
  constraint coincident L5 L11.start
  constraint coincident L7 L11.end
  constraint perpendicular L5 L11
extrude "Extrude5" cut sketch "Sketch6" against normal blind 6.8 contours L5 L6 L7 L11 bodies 1
extrude "Extrude6" add 1 faces at (135.9294, 68, 23.9589) along direction (0.991882, 0, 0.127164) blind 14.461 on bodies 1 bodies 1
sketch "Sketch7" plane through (-1.1004, 0, 8.5832) normal (-0.127164, 0, 0.991882) x (0, -1, 0)
  line L0 (-72, 137.8726) -> (-66, 137.8726)
  line L1 (-66, 137.8726) -> (-66, 152.3336)
  line L2 (-66, 152.3336) -> (-72, 152.3336)
  line L3 (-72, 152.3336) -> (-72, 137.8726)
  line L4 (-66, 152.3336) -> (-72.8279, 152.3336)
  line L5 (-72.8279, 152.3336) -> (-72.8279, 147.3336)
  line L6 (-72.8279, 147.3336) -> (-66, 147.3336)
  line L7 (-66, 147.3336) -> (-66, 152.3336)
  dimension "d30" = 5
  constraint horizontal L4
  constraint vertical L5
  constraint horizontal L6
  constraint vertical L7
  constraint coincident L1.end L2.start
  measures "d30" distance of L1.end L6.end
extrude "Extrude8" add sketch "Sketch7" along normal blind 30 contours L1 L2 L3 L4 L6 L7 bodies 1
sketch "Sketch8" plane through (151.0969, 0, 19.3714) normal (0.991882, 0, 0.127164) x (0, 1, 0)
  line L0 (72, 5.3918) -> (72, 38.6535)
  line L1 (72, 38.6535) -> (66, 38.6535)
  line L2 (66, 38.6535) -> (66, 5.3918)
  line L3 (66, 38.6535) -> (72, 38.6535)
  line L4 (72, 38.6535) -> (72, 33.6535)
  line L5 (72, 33.6535) -> (66, 33.6535)
  line L6 (66, 33.6535) -> (66, 38.6535)
  line L7 (66, 5.3918) -> (72, 5.3918)
  dimension "d33" = 5
  constraint horizontal L3
  constraint vertical L4
  constraint horizontal L5
  constraint vertical L6
  constraint coincident L1.end L2.start
  measures "d33" distance of L1.end L5.end
extrude "Extrude9" add sketch "Sketch8" along normal blind 72 contours L0 L1 L2 L3 L4 L5 L6 bodies 1
sketch "Sketch9" plane through (-4.2795, 0, 33.3803) normal (0.127164, 0, -0.991882) x (0, 1, 0)
  line L0 (66, 152.3336) -> (72, 152.3336)
  line L1 (72, 152.3336) -> (72, 224.3336)
  line L2 (72, 224.3336) -> (66, 224.3336)
  line L3 (66, 224.3336) -> (66, 152.3336)
  line L4 (72, 224.3336) -> (66, 224.3336)
  line L5 (66, 224.3336) -> (66, 219.3336)
  line L6 (66, 219.3336) -> (72, 219.3336)
  line L7 (72, 219.3336) -> (72, 224.3336)
  dimension "d36" = 5
  constraint horizontal L4
  constraint vertical L5
  constraint horizontal L6
  constraint vertical L7
  constraint coincident L3 L5.end
  constraint coincident L1.end L2.start
  measures "d36" distance of L1.end L6.end
extrude "Extrude10" add sketch "Sketch9" along normal blind 40 contours L1 L2 L3 L4 L5 L6 L7 bodies 1
sketch "Sketch10" plane through (0.807, 0, -6.295) normal (0.127164, 0, -0.991882) x (0, 1, 0)
  line L0 (72, 219.3336) -> (72, 224.3336)
  line L1 (72, 224.3336) -> (66, 224.3336)
  line L2 (66, 224.3336) -> (66, 219.3336)
  line L3 (66, 219.3336) -> (72, 219.3336)
  line L4 (66, 219.3336) -> (72.721, 219.3336)
  line L5 (66, 214.8336) -> (66, 219.3336)
  line L6 (72, 219.3336) -> (66, 219.3336)
  line L7 (66, 219.3336) -> (66, 214.8336)
  line L8 (66, 214.8336) -> (72, 214.8336)
  line L9 (72, 214.8336) -> (72, 219.3336)
  line L10 (66, 214.8336) -> (72, 214.8336)
  line L11 (72, 214.8336) -> (72, 209.8336)
  line L12 (72, 209.8336) -> (66, 209.8336)
  line L13 (66, 209.8336) -> (66, 214.8336)
  dimension "d40" = 6
  dimension "d41" = 4.5
  dimension "d56" = 5
  constraint horizontal L4
  constraint vertical L5
  constraint coincident L2.end L3.start
  constraint horizontal L6
  constraint vertical L7
  constraint horizontal L8
  constraint vertical L9
  constraint coincident L0.start L3.end
  constraint horizontal L10
  constraint vertical L11
  constraint horizontal L12
  constraint vertical L13
  measures "d40" distance of L0.start L2.end
  measures "d41" distance of L0.start L8.end
  measures "d56" distance of L5.start L12.end
extrude "Extrude11" add sketch "Sketch10" against normal blind 5 contours L3 L4 L5 L6 L7 L8 L9 L10 bodies 1
extrude "Extrude13" add sketch "Sketch3" along normal blind 6 contours L0 L2 L7 L9 L10 L11 L12 bodies 1
sketch "Sketch11" plane through (-0.6856, 0, 5.348) normal (0.127164, 0, -0.991882) x (0, 1, 0)
  line L0 (66, 114.3824) -> (72, 114.3824)
  line L1 (72, 114.3824) -> (72, 152.3336)
  line L2 (72, 152.3336) -> (66, 152.3336)
  line L3 (66, 152.3336) -> (66, 114.3824)
  line L4 (72, 152.3336) -> (65.9909, 152.3336)
  line L5 (65.9909, 152.3336) -> (65.9909, 147.3336)
  line L6 (65.9909, 147.3336) -> (72, 147.3336)
  line L7 (72, 147.3336) -> (72, 152.3336)
  dimension "d49" = 5
  constraint horizontal L4
  constraint vertical L5
  constraint horizontal L6
  constraint vertical L7
  constraint coincident L1.end L2.start
  measures "d49" distance of L1.end L6.end
extrude "Extrude14" add sketch "Sketch11" along normal blind 4 contours L1 L2 L3 L4 L6 L7 bodies 1
fillet "Fillet4" radius 1 2 edges at (113.5311, 69, 13.9421) (108.5717, 69, 13.3062) on bodies 1
fillet "Fillet5" radius 1 2 edges at (145.9605, 69, 20.116) (150.9199, 69, 20.7519) on bodies 1
extrude "Extrude15" add sketch "Sketch10" against normal blind 11 separate body contours L8 L10 L11 L12 L13 makes body 2
fillet "Fillet6" radius 2 4 edges at (223.3194, 69, 22.2322) (212.4977, 69, 31.9349) (207.5383, 69, 31.2991) (208.9371, 69, 20.3884) on bodies 1 2
sketch "Sketch12" plane through (0, 66, 0) normal (0, -1, 0) x (1, 0, 0)
  arc A0 (221.3356, 21.9779) -> (223.0651, 24.216) centre (221.0813, 23.9617) ccw
  line L0 (223.0651, 24.216) -> (217.597, 66.8669)
  line L1 (217.597, 66.8669) -> (141.2221, 57.0753)
  line L2 (141.2221, 57.0753) -> (145.037, 27.3188)
  line L3 (145.037, 27.3188) -> (135.6529, 26.1157)
  line L4 (135.6529, 26.1157) -> (130, 28)
  line L5 (130, 28) -> (87, 28)
  line L6 (87, 28) -> (87, 17)
  line L7 (87, 17) -> (65, 17)
  line L8 (65, 17) -> (65, 6)
  line L9 (65, 6) -> (70, 6)
  line L10 (70, 6) -> (70, 12)
  line L11 (70, 12) -> (92, 12)
  line L12 (92, 12) -> (92, 23)
  line L13 (92, 23) -> (98, 23)
  line L14 (98, 23) -> (98, 18)
  line L15 (98, 18) -> (107.8087, 19.2575)
  line L16 (107.8087, 19.2575) -> (108.4445, 14.2981)
  arc A1 (108.4445, 14.2981) -> (109.5636, 13.4334) centre (109.4364, 14.4253) ccw
  line L17 (109.5636, 13.4334) -> (112.5392, 13.8149)
  arc A2 (112.5392, 13.8149) -> (113.4039, 14.9339) centre (112.4121, 14.8068) ccw
  line L18 (113.4039, 14.9339) -> (112.7681, 19.8933)
  line L19 (112.7681, 19.8933) -> (145.4518, 24.0836)
  line L20 (145.4518, 24.0836) -> (145.8333, 21.1079)
  arc A3 (145.8333, 21.1079) -> (146.9524, 20.2432) centre (146.8252, 21.2351) ccw
  line L21 (146.9524, 20.2432) -> (149.928, 20.6247)
  arc A4 (149.928, 20.6247) -> (150.7927, 21.7437) centre (149.8008, 21.6166) ccw
  line L22 (150.7927, 21.7437) -> (146.8173, 52.7517)
  line L23 (146.8173, 52.7517) -> (213.2734, 61.2717)
  line L24 (213.2734, 61.2717) -> (217.7242, 26.5558)
  line L25 (217.7242, 26.5558) -> (213.2607, 25.9836)
  line L26 (213.2607, 25.9836) -> (213.8965, 21.0242)
  line L27 (213.8965, 21.0242) -> (221.3356, 21.9779)
  line L28 (98, 23) -> (98.6307, 18.0809)
  constraint coincident L13.end L14.start
  constraint coincident L15 L28.end
  constraint perpendicular L15 L28
extrude "Extrude16" cut sketch "Sketch12" against normal blind 8 contours L14 L15 L28 bodies 1
fillet "Fillet7" radius 2 2 edges at (87, 69, 28) (65, 69, 17) on bodies 1
fillet "Fillet8" radius 2 2 edges at (141.2221, 69, 57.0753) (217.597, 69, 66.8669) on bodies 1
fillet "Fillet8" radius 2.5 2 edges at (146.8173, 69, 52.7517) (213.2734, 69, 61.2717) on bodies 1
sketch "Sketch13" plane through (0, 66, 0) normal (0, -1, 0) x (1, 0, 0)
  arc A0 (217.8513, 64.8832) -> (215.6132, 66.6126) centre (215.8676, 64.6288) ccw
  line L0 (215.6132, 66.6126) -> (143.2059, 57.3296)
  arc A1 (143.2059, 57.3296) -> (141.4764, 55.0915) centre (143.4602, 55.3458) ccw
  line L1 (141.4764, 55.0915) -> (145.037, 27.3188)
  line L2 (145.037, 27.3188) -> (135.6529, 26.1157)
  line L3 (135.6529, 26.1157) -> (130, 28)
  line L4 (130, 28) -> (89, 28)
  arc A2 (89, 28) -> (87, 26) centre (89, 26) ccw
  line L5 (87, 26) -> (87, 17)
  line L6 (87, 17) -> (67, 17)
  arc A3 (67, 17) -> (65, 15) centre (67, 15) ccw
  line L7 (65, 15) -> (65, 6)
  line L8 (65, 6) -> (70, 6)
  line L9 (70, 6) -> (70, 12)
  line L10 (70, 12) -> (92, 12)
  line L11 (92, 12) -> (92, 23)
  line L12 (92, 23) -> (98, 23)
  line L13 (98, 23) -> (98.6307, 18.0809)
  line L14 (98.6307, 18.0809) -> (107.8087, 19.2575)
  line L15 (107.8087, 19.2575) -> (108.4445, 14.2981)
  arc A4 (108.4445, 14.2981) -> (109.5636, 13.4334) centre (109.4364, 14.4253) ccw
  line L16 (109.5636, 13.4334) -> (112.5392, 13.8149)
  arc A5 (112.5392, 13.8149) -> (113.4039, 14.9339) centre (112.4121, 14.8068) ccw
  line L17 (113.4039, 14.9339) -> (112.7681, 19.8933)
  line L18 (112.7681, 19.8933) -> (145.4518, 24.0836)
  line L19 (145.4518, 24.0836) -> (145.8333, 21.1079)
  arc A6 (145.8333, 21.1079) -> (146.9524, 20.2432) centre (146.8252, 21.2351) ccw
  line L20 (146.9524, 20.2432) -> (149.928, 20.6247)
  arc A7 (149.928, 20.6247) -> (150.7927, 21.7437) centre (149.8008, 21.6166) ccw
  line L21 (150.7927, 21.7437) -> (147.1353, 50.272)
  arc A8 (149.2971, 53.0696) -> (147.1353, 50.272) centre (149.615, 50.5899) ccw
  line L22 (149.2971, 53.0696) -> (210.7937, 60.9538)
  arc A9 (213.5913, 58.792) -> (210.7937, 60.9538) centre (211.1116, 58.4741) ccw
  line L23 (213.5913, 58.792) -> (217.7242, 26.5558)
  line L24 (217.7242, 26.5558) -> (213.2607, 25.9836)
  line L25 (213.2607, 25.9836) -> (213.8965, 21.0242)
  line L26 (213.8965, 21.0242) -> (221.3356, 21.9779)
  arc A10 (221.3356, 21.9779) -> (223.0651, 24.216) centre (221.0813, 23.9617) ccw
  line L27 (223.0651, 24.216) -> (217.8513, 64.8832)
  line L28 (180.0454, 57.0117) -> (180.6812, 52.0523)
  line L29 (180.6812, 52.0523) -> (213.9092, 56.3123)
  line L30 (180.6812, 52.0523) -> (147.4532, 47.7923)
  dimension "d69" = 5
  constraint midpoint L22 L28.start
  constraint perpendicular L22 L28
  constraint coincident L23 L29.end
  constraint perpendicular L23 L29
  constraint coincident L21 L30.end
  constraint perpendicular L21 L30
  measures "d69" distance of L28.start L28.end
extrude "Extrude17" add sketch "Sketch13" against normal blind 6 contours L22 A9 L23 L28 L29 | L21 A8 L22 L28 L30 bodies 1
sketch "Sketch14" plane through (0, 66, 0) normal (0, -1, 0) x (1, 0, 0)
  arc A0 (217.8513, 64.8832) -> (215.6132, 66.6126) centre (215.8676, 64.6288) ccw
  line L0 (215.6132, 66.6126) -> (143.2059, 57.3296)
  arc A1 (143.2059, 57.3296) -> (141.4764, 55.0915) centre (143.4602, 55.3458) ccw
  line L1 (141.4764, 55.0915) -> (145.037, 27.3188)
  line L2 (145.037, 27.3188) -> (135.6529, 26.1157)
  line L3 (135.6529, 26.1157) -> (130, 28)
  line L4 (130, 28) -> (89, 28)
  arc A2 (89, 28) -> (87, 26) centre (89, 26) ccw
  line L5 (87, 26) -> (87, 17)
  line L6 (87, 17) -> (67, 17)
  arc A3 (67, 17) -> (65, 15) centre (67, 15) ccw
  line L7 (65, 15) -> (65, 6)
  line L8 (65, 6) -> (70, 6)
  line L9 (70, 6) -> (70, 12)
  line L10 (70, 12) -> (92, 12)
  line L11 (92, 12) -> (92, 23)
  line L12 (92, 23) -> (98, 23)
  line L13 (98, 23) -> (98.6307, 18.0809)
  line L14 (98.6307, 18.0809) -> (107.8087, 19.2575)
  line L15 (107.8087, 19.2575) -> (108.4445, 14.2981)
  arc A4 (108.4445, 14.2981) -> (109.5636, 13.4334) centre (109.4364, 14.4253) ccw
  line L16 (109.5636, 13.4334) -> (112.5392, 13.8149)
  arc A5 (112.5392, 13.8149) -> (113.4039, 14.9339) centre (112.4121, 14.8068) ccw
  line L17 (113.4039, 14.9339) -> (112.7681, 19.8933)
  line L18 (112.7681, 19.8933) -> (145.4518, 24.0836)
  line L19 (145.4518, 24.0836) -> (145.8333, 21.1079)
  arc A6 (145.8333, 21.1079) -> (146.9524, 20.2432) centre (146.8252, 21.2351) ccw
  line L20 (146.9524, 20.2432) -> (149.928, 20.6247)
  arc A7 (149.928, 20.6247) -> (150.7927, 21.7437) centre (149.8008, 21.6166) ccw
  line L21 (150.7927, 21.7437) -> (147.4532, 47.7923)
  line L22 (147.4532, 47.7923) -> (213.9092, 56.3123)
  line L23 (213.9092, 56.3123) -> (217.7242, 26.5558)
  line L24 (217.7242, 26.5558) -> (213.2607, 25.9836)
  line L25 (213.2607, 25.9836) -> (213.8965, 21.0242)
  line L26 (213.8965, 21.0242) -> (221.3356, 21.9779)
  arc A8 (221.3356, 21.9779) -> (223.0651, 24.216) centre (221.0813, 23.9617) ccw
  line L27 (223.0651, 24.216) -> (217.8513, 64.8832)
  line L28 (213.9092, 56.3123) -> (213.2734, 61.2717) construction
  line L29 (213.2734, 61.2717) -> (141.8579, 52.1159) construction
  line L30 (141.8579, 52.1159) -> (218.2328, 61.9075)
  dimension "d72" = 5
  constraint coincident L22.end L23.start
  constraint perpendicular L22 L28
  constraint coincident L1 L29.end
  constraint perpendicular L1 L29
  constraint coincident L27 L30.end
  constraint perpendicular L27 L30
  measures "d72" distance of L22.end L28.end
extrude "Extrude18" cut sketch "Sketch14" against normal blind 10 contours A0 L0 A1 L1 L27 L30 bodies 1
fillet "Fillet9" radius 2 2 edges at (218.2328, 69, 61.9075) (141.8579, 69, 52.1159) on bodies 1
fillet "Fillet10" radius 1 2 edges at (213.9092, 69, 56.3123) (147.4532, 69, 47.7923) on bodies 1
combine "Combine1" operation add target body 2 tool bodies 1
sketch "Sketch15" plane through (0, 66, 0) normal (0, -1, 0) x (1, 0, 0)
  arc A0 (208.6828, 22.3721) -> (210.9209, 20.6427) centre (210.6666, 22.6265) ccw
  line L0 (210.9209, 20.6427) -> (221.3356, 21.9779)
  arc A1 (221.3356, 21.9779) -> (223.0651, 24.216) centre (221.0813, 23.9617) ccw
  line L1 (223.0651, 24.216) -> (218.4872, 59.9237)
  arc A2 (218.4872, 59.9237) -> (216.2491, 61.6532) centre (216.5034, 59.6694) ccw
  line L2 (216.2491, 61.6532) -> (143.8417, 52.3702)
  arc A3 (143.8417, 52.3702) -> (142.1123, 50.1321) centre (144.096, 50.3864) ccw
  line L3 (142.1123, 50.1321) -> (145.037, 27.3188)
  line L4 (145.037, 27.3188) -> (135.6529, 26.1157)
  line L5 (135.6529, 26.1157) -> (130, 28)
  line L6 (130, 28) -> (89, 28)
  arc A4 (89, 28) -> (87, 26) centre (89, 26) ccw
  line L7 (87, 26) -> (87, 17)
  line L8 (87, 17) -> (67, 17)
  arc A5 (67, 17) -> (65, 15) centre (67, 15) ccw
  line L9 (65, 15) -> (65, 6)
  line L10 (65, 6) -> (70, 6)
  line L11 (70, 6) -> (70, 12)
  line L12 (70, 12) -> (92, 12)
  line L13 (92, 12) -> (92, 23)
  line L14 (92, 23) -> (98, 23)
  line L15 (98, 23) -> (98.6307, 18.0809)
  line L16 (98.6307, 18.0809) -> (107.8087, 19.2575)
  line L17 (107.8087, 19.2575) -> (108.4445, 14.2981)
  arc A6 (108.4445, 14.2981) -> (109.5636, 13.4334) centre (109.4364, 14.4253) ccw
  line L18 (109.5636, 13.4334) -> (112.5392, 13.8149)
  arc A7 (112.5392, 13.8149) -> (113.4039, 14.9339) centre (112.4121, 14.8068) ccw
  line L19 (113.4039, 14.9339) -> (112.7681, 19.8933)
  line L20 (112.7681, 19.8933) -> (145.4518, 24.0836)
  line L21 (145.4518, 24.0836) -> (145.8333, 21.1079)
  arc A8 (145.8333, 21.1079) -> (146.9524, 20.2432) centre (146.8252, 21.2351) ccw
  line L22 (146.9524, 20.2432) -> (149.928, 20.6247)
  arc A9 (149.928, 20.6247) -> (150.7927, 21.7437) centre (149.8008, 21.6166) ccw
  line L23 (150.7927, 21.7437) -> (147.5803, 46.8004)
  arc A10 (148.4451, 47.9194) -> (147.5803, 46.8004) centre (148.5722, 46.9276) ccw
  line L24 (148.4451, 47.9194) -> (212.9174, 56.1851)
  arc A11 (214.0364, 55.3204) -> (212.9174, 56.1851) centre (213.0445, 55.1932) ccw
  line L25 (214.0364, 55.3204) -> (217.7242, 26.5558)
  line L26 (217.7242, 26.5558) -> (213.2607, 25.9836)
  line L27 (213.2607, 25.9836) -> (212.752, 29.9511)
  arc A12 (212.752, 29.9511) -> (210.514, 31.6806) centre (210.7683, 29.6968) ccw
  line L28 (210.514, 31.6806) -> (209.5221, 31.5534)
  arc A13 (209.5221, 31.5534) -> (207.7926, 29.3153) centre (209.7764, 29.5696) ccw
  line L29 (207.7926, 29.3153) -> (208.6828, 22.3721)
